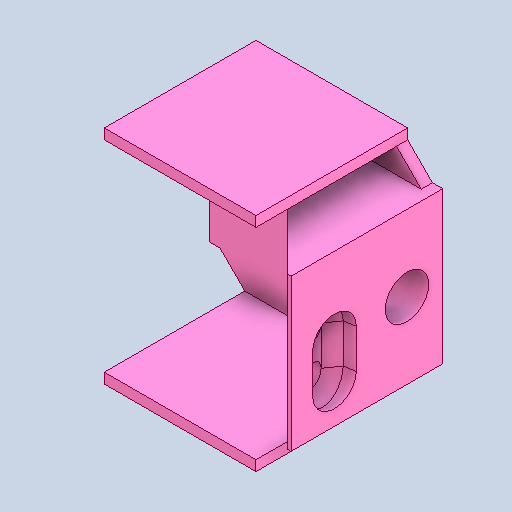
# Autodesk Inventor part: Mirror Base
Saved by Autodesk Inventor 2023.1 (Build 271208000, 208)
## iProperties
Created: 2022-08-09
Part Number: Mirror Base
Material: Generic
Document SubType Name: Modeling
Designer: xSibe
Density: 1 g/cm^3
Appearance: Plastic Pink
Author: xSibe
Autodesk Inventor part; units mm, degrees
ref_plane "YZ Plane" through (0, 0, 0) normal (1, 0, 0) x (0, 1, 0)
ref_plane "XZ Plane" through (0, 0, 0) normal (0, 1, 0) x (-1, 0, 0)
ref_plane "XY Plane" through (0, 0, 0) normal (0, 0, 1) x (1, 0, 0)
ref_plane "Work Plane1" through (-24.9, -24.9, 7.7) normal (0, 0, 1) x (1, 0, 0)
sketch "Sketch1" plane through (0, 0, 0) normal (0, 0, 1) x (0, 1, 0)
  circle A0 centre (20.9, 10) radius 1.875
  circle A1 centre (-20.9, 10) radius 1.875
  circle A2 centre (20.9, -10) radius 1.875
  circle A3 centre (-20.9, -10) radius 1.875
  circle A4 centre (-14.4, -20.8) radius 2.075
  circle A5 centre (14.4, -20.8) radius 2.075
  circle A6 centre (14.4, 20.8) radius 2.075
  circle A7 centre (-14.4, 20.8) radius 2.075
  line L0 (-16.9, -16.9) -> (-16.9, 16.9)
  line L1 (-16.9, 16.9) -> (16.9, 16.9)
  line L2 (16.9, 16.9) -> (16.9, -16.9)
  line L3 (16.9, -16.9) -> (-16.9, -16.9)
  line L4 (24.9, 17.05) -> (22.55, 17.05)
  line L5 (22.55, 17.05) -> (17.05, 22.55)
  line L6 (17.05, 22.55) -> (17.05, 24.9)
  line L7 (17.05, 24.9) -> (-17.05, 24.9)
  line L8 (-17.05, 24.9) -> (-17.05, 22.55)
  line L9 (-17.05, 22.55) -> (-22.55, 17.05)
  line L10 (-22.55, 17.05) -> (-24.9, 17.05)
  line L11 (-24.9, 17.05) -> (-24.9, -17.05)
  line L12 (-24.9, -17.05) -> (-22.55, -17.05)
  line L13 (-22.55, -17.05) -> (-17.05, -22.55)
  line L14 (-17.05, -22.55) -> (-17.05, -24.9)
  line L15 (-17.05, -24.9) -> (17.05, -24.9)
  line L16 (17.05, -24.9) -> (17.05, -22.55)
  line L17 (17.05, -22.55) -> (22.55, -17.05)
  line L18 (22.55, -17.05) -> (24.9, -17.05)
  line L19 (24.9, -17.05) -> (24.9, 17.05)
  line L20 (16.975, -24.825) -> (-16.975, -24.825)
  line L21 (-16.975, -24.825) -> (-16.975, -22.518934)
  line L22 (-16.975, -22.518934) -> (-22.518934, -16.975)
  line L23 (-22.518934, -16.975) -> (-24.825, -16.975)
  line L24 (-24.825, -16.975) -> (-24.825, 16.975)
  line L25 (-24.825, 16.975) -> (-22.518934, 16.975)
  line L26 (-22.518934, 16.975) -> (-16.975, 22.518934)
  line L27 (-16.975, 22.518934) -> (-16.975, 24.825)
  line L28 (-16.975, 24.825) -> (16.975, 24.825)
  line L29 (16.975, 24.825) -> (16.975, 22.518934)
  line L30 (16.975, 22.518934) -> (22.518934, 16.975)
  line L31 (22.518934, 16.975) -> (24.825, 16.975)
  line L32 (24.825, 16.975) -> (24.825, -16.975)
  line L33 (24.825, -16.975) -> (22.518934, -16.975)
  line L34 (22.518934, -16.975) -> (16.975, -22.518934)
  line L35 (16.975, -22.518934) -> (16.975, -24.825)
  dimension "d5" = 0.075
  constraints: 32 end point, 15 other
  measures "d5" distance between parallel lines of L15 L20
extrude "Extrusion1" add sketch "Sketch1" along normal blind 2.5 from surface at 7.7 contours A0 | A1 | A2 | A3 | A4 | A5 | A6 | A7 | L0 L1 L2 L3 | L20 L21 L22 L23 L24 L25 L26 L27 L28 L29 L30 L31 L32 L33 L34 L35
sketch "Sketch2" plane through (0, 0, 0) normal (0, 1, 0) x (-1, 0, 0)
  line L0 (16.975, 10.2) -> (-16.975, 10.2)
  line L1 (-16.975, 7.7) -> (-16.975, 10.2)
  line L2 (16.975, 7.7) -> (-16.975, 7.7)
  line L3 (16.975, 7.7) -> (16.975, 10.2)
  line L4 (16.975, 7.7) -> (-16.975, 41.65)
  line L5 (16.975, 7.7) -> (64.98755, 7.7) construction
  line L6 (-16.975, 41.65) -> (-16.975, 10.2)
  line L7 (-20.510534, 41.65) -> (10.939466, 10.2)
  line L8 (7.403932, 10.2) -> (-24.046068, 41.65)
  line L9 (-19.475, 12.7) -> (19.475, 12.7)
  line L10 (19.475, 12.7) -> (19.475, 5.2)
  line L11 (19.475, 5.2) -> (-19.475, 5.2)
  line L12 (-19.475, 5.2) -> (-19.475, 12.7)
  line L13 (-16.975, 41.65) -> (-24.825, 41.65)
  line L14 (-24.825, 41.65) -> (-24.825, 10.2)
  line L15 (-24.825, 10.2) -> (-16.975, 10.2)
  line L16 (-16.975, 10.2) -> (-16.975, 41.65)
  point P0 (0, 0)
  point P1 (14.475, 10.2)
  point P2 (-16.975, 38.114466)
  point P3 (-16.975, 34.578932)
  point P4 (8.439466, 12.7)
  point P5 (11.975, 12.7)
  point P6 (-19.475, 10.2)
  point P7 (-16.975, 12.7)
  point P8 (-16.975, 10.2)
  dimension "d6" = 135
  dimension "d9" = 2.5
  dimension "d10" = 2.5
  dimension "d13" = 2.5
  constraints: 26 end point, 8 point on line, 2 horizontal, 2 parallel, 2 perpendicular, 1 equal length, 3 other
  measures "d6" angle of L5 L4
  measures "d9" distance between parallel lines of L4 L7
  measures "d10" distance between parallel lines of L7 L8
  measures "d13" distance between parallel lines of L0 L9
extrude "Extrusion2" add sketch "Sketch2" along normal mid plane 33.95 contours L7 L9 L4 L0 | L0 L8 L9 L7 | L0 L6 L9 L8 | L9 L8 L6 L7 | L7 L6 L4 L9 | L15 L12 L9 L6 | L9 L6 L8 | L7 L13 L6 | L6 L8 L13 L7 | L9 L12 L15 L14 L13 L8 L6
extrude "Extrusion3" cut sketch "Sketch2" along normal mid plane 33.95 contours L7 L9 L4 L0 | L0 L8 L9 L7 | L9 L8 L6 L7 | L7 L13 L6 | L6 L8 L13 L7
ref_plane "Work Plane2" through (24.825, 0, 41.65) normal (0.9848078, 0, -0.1736482) x (0, 1, 0)
sketch "Sketch3" plane through (20.764317, -15, 18.620724) normal (0.9848078, 0, -0.1736482) x (-0.1736482, 0, -0.9848078)
  line L0 (10.901958, -1.975) -> (10.901958, 31.975)
  line L1 (-18.539581, 15) -> (10.901958, 15)
  line L2 (6.181189, 6.25) -> (-13.818811, 6.25)
  line L3 (-13.818811, 6.25) -> (-13.818811, 23.75)
  line L4 (-13.818811, 23.75) -> (6.181189, 23.75)
  line L5 (6.181189, 23.75) -> (6.181189, 6.25)
  line L6 (6.181189, 6.25) -> (-13.818811, 23.75) construction
  line L7 (-13.818811, 6.25) -> (6.181189, 23.75) construction
  circle A0 centre (-13.818811, 6.25) radius 2.3
  circle A1 centre (-13.818811, 6.25) radius 4.8
  line L8 (-3.818811, 15) -> (-3.818811, 6.25)
  line L9 (-3.818811, 10.625) -> (-13.818811, 10.625)
  line L10 (-8.818811, 10.625) -> (-8.818811, 6.25)
  circle A2 centre (-13.818811, 15) radius 2.3
  circle A3 centre (-13.818811, 15) radius 4.8
  circle A4 centre (-3.818811, 15) radius 4.8
  circle A5 centre (-3.818811, 15) radius 2.3
  line L11 (-18.618811, 6.25) -> (-18.618811, 15)
  line L12 (-9.018811, 15) -> (-9.018811, 6.25)
  line L13 (-18.539581, -1.975) -> (-18.539581, 31.975)
  line L14 (10.901958, -1.975) -> (-18.539581, -1.975)
  line L15 (-18.539581, 31.975) -> (10.901958, 31.975)
  point P0 (21.943519, 15)
  dimension "d16" = 20
  dimension "d17" = 17.5
  dimension "d18" = 4.6
  dimension "d19" = 2.5
  constraints: 24 end point, 8 midpoint, 6 centre point, 5 point on line, 4 point on circle, 3 perpendicular, 2 parallel, 1 coincident, 1 horizontal, 1 symmetric about line, 1 tangent, 4 other
  measures "d16" distance of L3.end L4.end
  measures "d17" distance of L2.end L3.end
  measures "d18" diameter of A0
  measures "d19" radial gap between concentric circles of A0 A1
extrude "Extrusion4" cut sketch "Sketch3" along normal mid plane 50 contours A0 L3 L2 | L2 L3 A0 | A2 L1 L3 | L3 L1 A2 | L1 L3 A2 | A2 L3 L1
extrude "Extrusion5" cut sketch "Sketch3" along normal blind 4.25 and the other way blind 2.5 contours L13 A1 A3 L3 A0 L2 | A1 L13 | L11 A3 L13 A1 | L2 A0 L3 A3 A1 | A1 L9 L12 | L13 A3 A1 | L13 A3 | A3 L3 A2 L1 L13 | A0 L3 L2 | L2 L3 A0 | L9 L3 A1 | A3 L12 L9 | A3 L3 L9 | A1 L3 A2 L1 A3 | A3 L13 L1 A2 L3 A1 | A1 L3 A3 | A3 L1 A2 L3 | A2 L1 L3 | L3 L1 A2 | L1 L3 A2 | A2 L3 L1
sketch "Sketch4" plane through (17.89206, 0, 2.331341) normal (0.9848078, 0, -0.1736482) x (0, 1, 0)
  line L0 (-16.975, 5.638714) -> (16.975, 5.638714)
  circle A0 centre (0, 14.388714) radius 2.3
  circle A1 centre (0, 14.388714) radius 4.8
  line L1 (-16.975, 35.080253) -> (16.975, 35.080253)
  line L2 (0, 5.638714) -> (0, 14.388714)
  line L3 (-16.975, 5.638714) -> (-16.975, 35.080253)
  line L4 (16.975, 35.080253) -> (16.975, 5.638714)
  circle A2 centre (-31.975, 20.359484) radius 2.5875
  line L5 (-31.975, 20.359484) -> (-16.975, 20.359484)
  line L6 (-16.975, 6.490989) -> (-16.975, 39.925212)
  point P0 (0, -5.164484)
  dimension "d25" = 4.6
  dimension "d26" = 2.5
  dimension "d37" = 8.75
  dimension "d117" = 5.175
  dimension "d118" = 15
  constraints: 4 end point, 3 centre point, 2 midpoint, 1 coincident, 1 perpendicular, 1 vertical
  measures "d25" diameter of A0
  measures "d26" radial gap between concentric circles of A0 A1
  measures "d37" distance of L2.start L2.end
  measures "d117" diameter of A2
  measures "d118" distance of L5.start L5.end
extrude "Extrusion6" cut sketch "Sketch4" along normal mid plane 100 contours A0
extrude "Extrusion7" cut sketch "Sketch4" along normal blind 15 and the other way blind 12.5 contours A0 | A1
sketch "Sketch7" plane through (-3.587512, 0, 17.551954) normal (0, 1, 0) x (-0.7071068, 0, -0.7071068)
  line L0 (-20.509007, 0) -> (-26.12457, 0)
  line L1 (-1.012297, 0) -> (-6.62786, 0)
  line L2 (0.738221, 2.5) -> (-1.012297, 0)
  line L3 (-4.877342, 2.5) -> (0.738221, 2.5)
  line L4 (-4.877342, 2.5) -> (-6.62786, 0)
  line L5 (-18.758488, 2.5) -> (-20.509007, 0)
  line L6 (-24.374051, 2.5) -> (-18.758488, 2.5)
  line L7 (-24.374051, 2.5) -> (-26.12457, 0)
  line L8 (-3.820079, 0) -> (-4.070079, 0)
  line L9 (-23.316788, 0) -> (-23.566788, 0)
  line L10 (-1.744777, -1.42544) -> (-6.742677, -0.544176)
  line L11 (-6.742677, -0.544176) -> (-6.39538, 1.42544)
  line L12 (-6.39538, 1.42544) -> (-1.397481, 0.544176)
  line L13 (-1.397481, 0.544176) -> (-1.744777, -1.42544)
  line L14 (-1.744777, -1.42544) -> (-6.39538, 1.42544) construction
  line L15 (-6.742677, -0.544176) -> (-1.397481, 0.544176) construction
  line L16 (-1.744777, -1.42544) -> (3.330223, -1.42544) construction
  line L17 (-21.241487, -1.42544) -> (-26.239386, -0.544176)
  line L18 (-26.239386, -0.544176) -> (-25.89209, 1.42544)
  line L19 (-25.89209, 1.42544) -> (-20.894191, 0.544176)
  line L20 (-20.894191, 0.544176) -> (-21.241487, -1.42544)
  line L21 (-21.241487, -1.42544) -> (-25.89209, 1.42544) construction
  line L22 (-26.239386, -0.544176) -> (-20.894191, 0.544176) construction
  line L23 (-21.241487, -1.42544) -> (-16.166487, -1.42544) construction
  line L24 (-27.108829, 3.163124) -> (-27.97707, -1.760915)
  line L25 (-27.97707, -1.760915) -> (-20.024748, -3.163124)
  line L26 (-20.024748, -3.163124) -> (-19.156507, 1.760915)
  line L27 (-19.156507, 1.760915) -> (-27.108829, 3.163124)
  line L28 (-7.61212, 3.163124) -> (-8.480361, -1.760915)
  line L29 (-8.480361, -1.760915) -> (-0.528038, -3.163124)
  line L30 (-0.528038, -3.163124) -> (0.340203, 1.760915)
  line L31 (0.340203, 1.760915) -> (-7.61212, 3.163124)
  line L32 (-1.012297, 0) -> (0.029706, 0)
  line L33 (-20.509007, 0) -> (-19.467004, 0)
  line L34 (-1.744777, -1.42544) -> (0.029706, 0)
  line L35 (-21.241487, -1.42544) -> (-19.467004, 0)
  line L36 (-26.12457, 0) -> (-27.666573, 0)
  line L37 (-6.62786, 0) -> (-8.169864, 0)
  line L38 (-6.742677, -0.544176) -> (-8.169864, 0)
  line L39 (-26.239386, -0.544176) -> (-27.666573, 0)
  point P0 (-1.493434, 0)
  point P1 (-6.646724, 0)
  point P2 (-26.143433, 0)
  point P3 (-20.990143, 0)
  dimension "d70" = 0.25
  dimension "d71" = 0.25
  dimension "d72" = 5.075
  dimension "d73" = 170
  dimension "d74" = 2
  dimension "d75" = 5.075
  dimension "d76" = 170
  dimension "d77" = 2
  dimension "d78" = 1.5
  dimension "d79" = 1.5
  constraints: 64 end point, 8 parallel, 8 point on line, 6 midpoint, 5 perpendicular, 4 horizontal, 2 equal length, 6 other
  measures "d70" distance of L8.start L8.end
  measures "d71" distance of L9.start L9.end
  measures "d72" distance of L10.start L10.end
  measures "d73" angle of L16 L10
  measures "d74" distance of L10.end L11.end
  measures "d75" distance of L17.start L17.end
  measures "d76" angle of L23 L17
  measures "d77" distance of L17.end L18.end
  measures "d78" distance between parallel lines of L18 L24
  measures "d79" distance between parallel lines of L11 L28
extrude "Extrusion10" add sketch "Sketch7" along normal mid plane 33.95 contours L0 L7 L19 L20 | L20 L19 L7 L6 L27 L5 L0 | L27 L6 L5 | L1 L4 L12 L13 | L13 L12 L4 L3 L31 L2 L1 | L31 L3 L2
extrude "Extrusion11" cut sketch "Sketch7" along normal mid plane 5.075 contours L0 L20 L17 L18 L36 | L0 L7 L19 L20 | L36 L18 L19 L7 | L1 L13 L10 L11 L37 | L1 L4 L12 L13 | L37 L11 L12 L4
sketch "Sketch8" plane through (13.713022, -15.0375, 36.868364) normal (0.819152, 0, -0.5735764) x (-0.5735764, 0, -0.819152)
  line L0 (0, 12.5) -> (0, 17.575) projected
  line L1 (5.075, 17.575) -> (5.075, 12.5) projected
  line L2 (0, 12.5) -> (5.075, 12.5) projected
  line L3 (5.075, 17.575) -> (0, 17.575) projected
  line L4 (2.5375, 12.5) -> (2.5375, 17.575)
  circle A0 centre (2.5375, 15.0375) radius 2.5375
  circle A1 centre (2.5375, 15.0375) radius 4.0375
  circle A2 centre (2.5375, 6.2875) radius 4.0375
  circle A3 centre (2.5375, 6.2875) radius 2.5375
  line L5 (-1.5, 15.0375) -> (-1.5, 6.2875)
  line L6 (6.575, 15.0375) -> (6.575, 6.2875)
  point P0 (38.066262, 15.0375)
  dimension "d86" = 5.075
  dimension "d87" = 1.5
  dimension "d90" = 8.75
  constraints: 6 end point, 4 centre point, 4 point on circle, 4 tangent, 3 midpoint, 1 vertical, 3 other
  measures "d86" diameter of A0
  measures "d87" radial gap between concentric circles of A0 A1
  measures "d90" distance of A0.centre A3.centre
extrude "Extrusion12" cut sketch "Sketch8" along normal blind 1.5 contours A0 L4 | L4 A0 | A3
extrude "Extrusion13" add sketch "Sketch8" along normal blind 1.5 contours L0 A0 L2 | L0 L3 A0 | A0 L1 L2 | L3 L1 A0 | A1 | L6 A2 L5 A1 | A2
sketch "Sketch9" plane through (-0.073234, -2.5375, 23.082109) normal (0.819152, 0, -0.5735764) x (-0.5735764, 0, -0.819152)
  line L0 (0, 0) -> (0, 5.075) projected
  line L1 (0, 0) -> (5.075, 0) projected
  line L2 (5.075, 5.075) -> (5.075, 0) projected
  line L3 (5.075, 5.075) -> (0, 5.075) projected
  line L4 (2.5375, 0) -> (2.5375, 5.075)
  circle A0 centre (2.5375, 2.5375) radius 2.5375
  circle A1 centre (2.5375, 2.5375) radius 4.0375
  point P0 (18.865751, 2.5375)
  dimension "d99" = 5.075
  dimension "d100" = 1.5
  constraints: 3 midpoint, 2 centre point, 2 end point
  measures "d99" diameter of A0
  measures "d100" radial gap between concentric circles of A0 A1
extrude "Extrusion14" add sketch "Sketch9" along normal blind 1.5 contours L0 A0 L1 | L0 L3 A0 | A0 L2 L1 | L3 L2 A0 | A1
chamfer "Chamfer1" distance 1.21 angle 45 3 edges at (11.9583, -12.4749, 33.0978) (-1.8279, 3.7249, 19.3115) (-1.8279, -3.7249, 19.3115)
sketch "Sketch10" plane through (0, 0, 0) normal (0, 1, 0) x (-1, 0, 0)
  line L0 (-11.176401, 30.630525) -> (-15.112756, 36.252222)
  line L1 (-11.168912, 30.623176) -> (-11.176401, 30.630525)
  line L2 (-15.112756, 36.252222) -> (-9.322139, 30.461605)
  line L3 (22.518934, 10.2) -> (24.825, 10.2)
  line L4 (24.825, 7.7) -> (24.825, 10.2)
  line L5 (22.518934, 7.7) -> (24.825, 7.7)
  line L6 (22.518934, 7.7) -> (22.518934, 10.2)
  line L7 (16.975, 10.2) -> (22.518934, 10.2)
  line L8 (22.518934, 7.7) -> (22.518934, 10.2)
  line L9 (16.975, 7.7) -> (22.518934, 7.7)
  line L10 (16.975, 7.7) -> (16.975, 10.2)
  line L11 (-16.975, 10.2) -> (16.975, 10.2)
  line L12 (16.975, 7.7) -> (16.975, 10.2)
  line L13 (-16.975, 7.7) -> (16.975, 7.7)
  line L14 (-16.975, 7.7) -> (-16.975, 10.2)
  line L15 (-22.518934, 10.2) -> (-16.975, 10.2)
  line L16 (-16.975, 7.7) -> (-16.975, 10.2)
  line L17 (-22.518934, 7.7) -> (-16.975, 7.7)
  line L18 (-22.518934, 7.7) -> (-22.518934, 10.2)
  line L19 (-11.168912, 30.623176) -> (-9.322139, 30.461605)
  line L20 (7.403932, 10.2) -> (-24.046068, 41.65)
  line L21 (-24.046068, 41.65) -> (-24.825, 41.65)
  line L22 (-24.825, 7.7) -> (-24.825, 41.65)
  line L23 (-22.518934, 7.7) -> (-24.825, 7.7)
  line L24 (-22.518934, 10.2) -> (-22.518934, 7.7)
  line L25 (7.403932, 10.2) -> (-22.518934, 10.2)
  line L26 (11.975, 12.7) -> (-16.975, 41.65)
  line L27 (-16.975, 41.65) -> (-16.975, 38.114466)
  line L28 (-16.975, 38.114466) -> (8.439466, 12.7)
  line L29 (8.439466, 12.7) -> (11.975, 12.7)
  line L30 (-1.326501, 22.465967) -> (2.609854, 16.844269)
  line L31 (2.609854, 16.844269) -> (2.609854, 16.844269)
  line L32 (2.609854, 16.844269) -> (-1.326501, 22.465967)
  line L33 (-1.326501, 22.465967) -> (-1.326501, 22.465967)
  line L34 (2.609854, 16.844269) -> (4.456782, 16.682684)
  line L35 (-11.168912, 30.623176) -> (2.609854, 16.844269)
  line L36 (2.609854, 16.844269) -> (8.439466, 12.7)
  line L37 (-16.975, 38.114466) -> (8.439466, 12.7)
  line L38 (8.439466, 12.7) -> (7.068649, 11.329183)
  line L39 (7.068649, 11.329183) -> (-18.345817, 36.743649)
  line L40 (-18.345817, 36.743649) -> (-16.975, 38.114466)
  point P0 (0, 0)
  constraints: 14 end point, 3 equal length, 1 perpendicular, 1 point on line
extrude "Extrusion15" cut sketch "Sketch10" along normal mid plane 33.95 contours L1 L35 L36 L38 L39 L40 L28 L0 | L0 L2 L19 L1 | L28 L27 L26 L29 L2 | L19 L28 L30 L35 | L30 L28 L34 | L34 L28 L36
chamfer "Chamfer3" distance 2.5 angle 45 4 edges at (20.6999, 4.8, 32.6641) (19.8664, -4.375, 27.937) (20.6999, -13.55, 32.6641) (21.5335, -4.375, 37.3911)
sketch "Sketch11" plane through (-16.975, 24.825, 10.2) normal (0, 0, 1) x (1, 0, 0)
  line L0 (9.571068, -7.85) -> (39.493934, -7.85)
  line L1 (33.95, -2.306066) -> (39.493934, -7.85)
  line L2 (33.95, 0) -> (33.95, -2.306066)
  line L3 (0, 0) -> (33.95, 0)
  line L4 (0, -2.306066) -> (0, 0)
  line L5 (-5.543934, -7.85) -> (0, -2.306066)
  line L6 (-7.85, -7.85) -> (-5.543934, -7.85)
  line L7 (-7.85, -41.8) -> (-7.85, -7.85)
  line L8 (-5.543934, -41.8) -> (-7.85, -41.8)
  line L9 (0, -47.343934) -> (-5.543934, -41.8)
  line L10 (0, -49.65) -> (0, -47.343934)
  line L11 (33.95, -49.65) -> (0, -49.65)
  line L12 (33.95, -47.343934) -> (33.95, -49.65)
  line L13 (39.493934, -41.8) -> (33.95, -47.343934)
  line L14 (39.493934, -41.8) -> (9.571068, -41.8)
  line L15 (33.95, -49.65) -> (0, -49.65)
  line L16 (0, -49.65) -> (0, -47.343934)
  line L17 (0, -47.343934) -> (33.95, -47.343934)
  line L18 (33.95, -47.343934) -> (33.95, -49.65)
  line L19 (33.95, 0) -> (0, 0)
  line L20 (0, 0) -> (0, -2.306066)
  line L21 (0, -2.306066) -> (33.95, -2.306066)
  line L22 (33.95, -2.306066) -> (33.95, 0)
  line L23 (41.8, -41.8) -> (41.021068, -41.8)
  line L24 (41.8, -41.8) -> (41.8, -7.85)
  line L25 (41.021068, -7.85) -> (41.8, -7.85)
  line L26 (41.021068, -7.85) -> (41.021068, -41.8)
  line L27 (9.571068, -41.8) -> (9.571068, -7.85)
  point P0 (16.975, -24.825)
  constraints: 16 end point, 4 parallel, 2 horizontal, 2 perpendicular
extrude "Extrusion16" add sketch "Sketch11" along normal blind 31.45 contours L21 L4 L3 L2 | L12 L11 L10 L17
body "Solid1"
